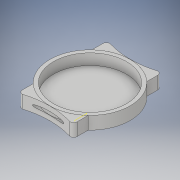
# Autodesk Inventor part: watchBodyOne
Saved by Autodesk Inventor 2019 (Build 230136000, 136)
## iProperties
Created: 2019-10-08
Part Number: watchBodyOne
Material: Generic
Document SubType Name: Modeling
Designer: Derek
Density: 1 g/cm^3
Appearance: Default
Author: Derek
Autodesk Inventor part; units mm, degrees
ref_plane "YZ Plane" through (0, 0, 0) normal (1, 0, 0) x (0, 1, 0)
ref_plane "XZ Plane" through (0, 0, 0) normal (0, 1, 0) x (-1, 0, 0)
ref_plane "XY Plane" through (0, 0, 0) normal (0, 0, 1) x (1, 0, 0)
sketch "Sketch1" plane through (0, 0, 0) normal (0, 1, 0) x (-1, 0, 0)
  circle A0 centre (0, 0) radius 22
  arc A1 (-13.723822, -17.194671) -> (13.723822, -17.194671) centre (0, 0) ccw
  dimension "d0" = 44
  dimension "d11" = 13.72382
  constraints: 4 point on circle, 2 centre point, 1 coincident, 1 concentric
  measures "d0" diameter of A0
  measures "d11" horizontal distance of point (0, 0) A0.start
sketch "Sketch1 outline for Main Base" plane through (0, 0, 0) normal (0, 1, 0) x (-1, 0, 0)
  circle A0 centre (0, 0) radius 22
extrude "Main Base" add sketch "Sketch1 outline for Main Base" along normal blind 7
sketch "Sketch5" plane through (0, 7, 0) normal (0, 1, 0) x (1, 0, 0)
  circle A0 centre (0, 0) radius 20
  dimension "d8" = 40
  constraints: 1 centre point, 1 coincident
  measures "d8" diameter of A0
sketch "Sketch5 outline for Hole" plane through (0, 7, 0) normal (0, 1, 0) x (1, 0, 0)
  circle A0 centre (0, 0) radius 20
extrude "Hole" cut sketch "Sketch5 outline for Hole" against normal blind 6
sketch "Sketch8" plane through (0, 0, 0) normal (0, -1, 0) x (1, 0, 0)
  arc A0 (-11.587375, -18.701143) -> (11.587375, -18.701143) centre (0, 0) ccw
  line L0 (-15.045316, -16.051121) -> (-15.045316, -22.025733)
  line L1 (15.045316, -16.051121) -> (15.045316, -22.025733)
  arc A1 (-15.045316, -16.051121) -> (15.045316, -16.051121) centre (0, 0) ccw
  arc A2 (-15.045316, -22.025733) -> (-13.045316, -24.025733) centre (-13.045316, -22.025733) ccw
  arc A3 (13.045316, -24.025733) -> (15.045316, -22.025733) centre (13.045316, -22.025733) ccw
  line L2 (-15.045053, -16.05136) -> (-15.045053, -22.025973)
  arc A4 (-15.045053, -22.025973) -> (-13.045053, -24.025973) centre (-13.045053, -22.025973) ccw
  arc A5 (13.045579, -24.025973) -> (15.045579, -22.025973) centre (13.045579, -22.025973) ccw
  line L3 (15.045579, -16.05136) -> (15.045579, -22.025973)
  arc A6 (-15.045053, -16.05136) -> (15.045579, -16.05136) centre (0.000263, -0.000239) ccw
  arc A7 (13.045579, -24.025973) -> (-13.045053, -24.025973) centre (0.000263, -66.847526) ccw
  point P0 (0, 0)
  point P1 (0, 0)
  constraints: 16 point on circle, 8 centre point, 8 end point
sketch "Sketch8 outline for Top Band" plane through (0, 0, 0) normal (0, -1, 0) x (1, 0, 0)
  line L0 (15.045579, -16.05136) -> (15.045579, -22.025973)
  arc A0 (15.045579, -22.025973) -> (13.045579, -24.025973) centre (13.045579, -22.025973) cw
  arc A1 (13.045579, -24.025973) -> (-13.045053, -24.025973) centre (0.000263, -66.847526) ccw
  arc A2 (-13.045053, -24.025973) -> (-15.045053, -22.025973) centre (-13.045053, -22.025973) cw
  line L1 (-15.045053, -22.025973) -> (-15.045053, -16.05136)
  arc A3 (-15.045053, -16.05136) -> (15.045579, -16.05136) centre (0.000263, -0.000239) ccw
extrude "Top Band" add sketch "Sketch8 outline for Top Band" against normal blind 7
sketch "Sketch11" plane through (0, 0, 0) normal (0, -1, 0) x (1, 0, 0)
  arc A0 (11.587375, 18.701143) -> (-11.587375, 18.701143) centre (0, 0) ccw
  line L0 (-15.045316, 16.051121) -> (-15.045316, 22.025733)
  line L1 (15.045316, 16.051121) -> (15.045316, 22.025733)
  arc A1 (15.045316, 16.051121) -> (-15.045316, 16.051121) centre (0, 0) ccw
  arc A2 (-13.045316, 24.025733) -> (-15.045316, 22.025733) centre (-13.045316, 22.025733) ccw
  arc A3 (15.045316, 22.025733) -> (13.045316, 24.025733) centre (13.045316, 22.025733) ccw
  line L2 (-15.045053, 16.05136) -> (-15.045053, 22.025973)
  arc A4 (-13.045053, 24.025973) -> (-15.045053, 22.025973) centre (-13.045053, 22.025973) ccw
  arc A5 (15.045579, 22.025973) -> (13.045579, 24.025973) centre (13.045579, 22.025973) ccw
  line L3 (15.045579, 16.05136) -> (15.045579, 22.025973)
  arc A6 (15.045579, 16.05136) -> (-15.045053, 16.05136) centre (0.000263, 0.000239) ccw
  arc A7 (-13.045053, 24.025973) -> (13.045579, 24.025973) centre (0.000263, 66.847526) ccw
  point P0 (0, 0)
  dimension "d27" = 2
  dimension "d28" = 2
  constraints: 16 point on circle, 8 centre point, 8 end point, 4 tangent, 4 vertical, 2 equal radius
  measures "d27" radius of A2
  measures "d28" radius of A4
sketch "Sketch11 outline for Bottom Band" plane through (0, 0, 0) normal (0, -1, 0) x (1, 0, 0)
  arc A0 (13.045579, 24.025973) -> (-13.045053, 24.025973) centre (0.000263, 66.847526) cw
  arc A1 (15.045579, 22.025973) -> (13.045579, 24.025973) centre (13.045579, 22.025973) ccw
  line L0 (15.045579, 16.05136) -> (15.045579, 22.025973)
  arc A2 (-15.045053, 16.05136) -> (15.045579, 16.05136) centre (0.000263, 0.000239) cw
  line L1 (-15.045053, 22.025973) -> (-15.045053, 16.05136)
  arc A3 (-13.045053, 24.025973) -> (-15.045053, 22.025973) centre (-13.045053, 22.025973) ccw
extrude "Bottom Band" add sketch "Sketch11 outline for Bottom Band" against normal blind 7
ref_plane "Work Plane2" through (14.045579, 0, 22.025973) normal (1, 0, 0) x (0, 0, -1)
sketch "Sketch14" plane through (14.045579, 0, 22.025973) normal (1, 0, 0) x (0, 0, -1)
  line L0 (0, 0) -> (0, 7) projected
  circle A0 centre (0, 3.5) radius 0.9
  point P0 (22.025973, 0)
  dimension "d38" = 1.8
  constraints: 1 centre point, 1 midpoint
  measures "d38" diameter of A0
sketch "Sketch14 outline for Extrusion11" plane through (14.045579, 0, 22.025973) normal (1, 0, 0) x (0, 0, -1)
  circle A0 centre (0, 3.5) radius 0.9
extrude "Extrusion11" cut sketch "Sketch14 outline for Extrusion11" against normal blind 28.2
sketch "Sketch15" plane through (14.045579, 0, 22.025973) normal (1, 0, 0) x (0, 0, -1)
  line L0 (44.10894, 7) -> (44.10894, 0)
  circle A0 centre (44.10894, 3.5) radius 0.9
  point P0 (22.025973, 0)
  dimension "d41" = 1.8
  constraints: 1 centre point, 1 midpoint
  measures "d41" diameter of A0
sketch "Sketch15 outline for Extrusion12" plane through (14.045579, 0, 22.025973) normal (1, 0, 0) x (0, 0, -1)
  circle A0 centre (44.10894, 3.5) radius 0.9
extrude "Extrusion12" cut sketch "Sketch15 outline for Extrusion12" against normal blind 28.2
body "Solid1"
